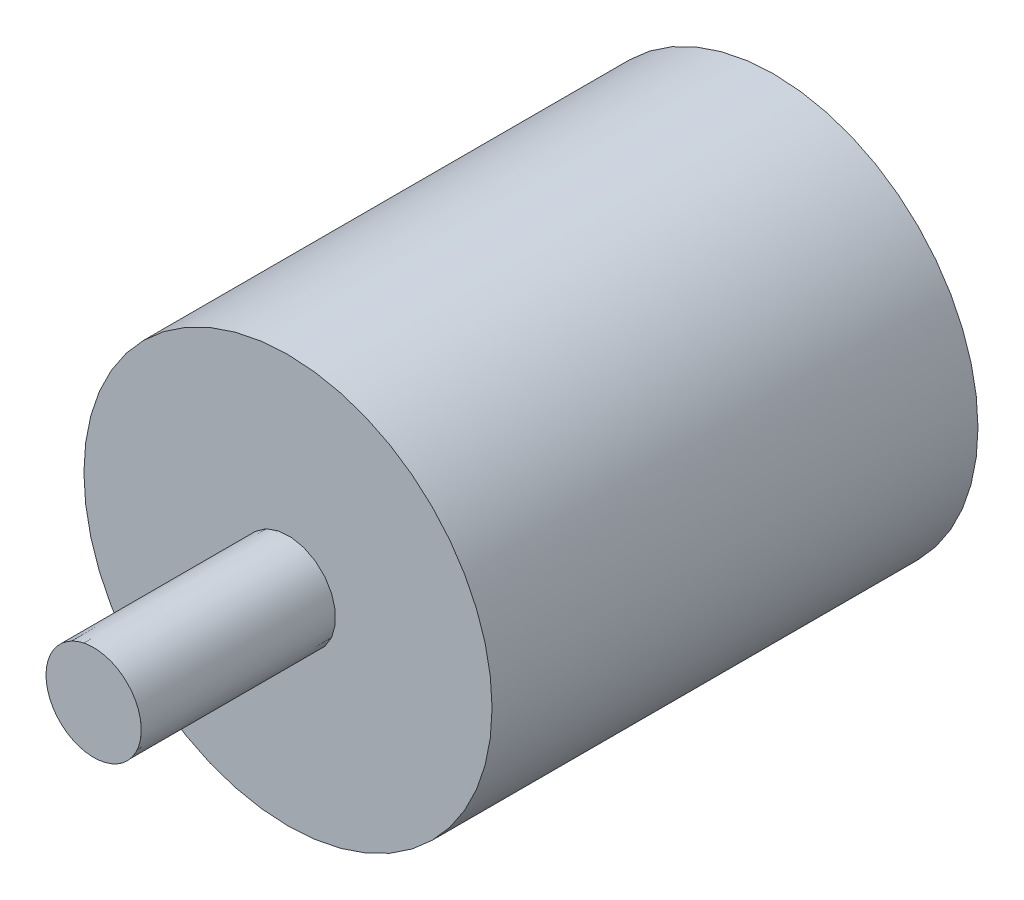
# Autodesk Inventor part: motor
Saved by Autodesk Inventor 2022 (Build 260153000, 153)
## iProperties
Created: 2022-03-03
Part Number: motor
Material: Generic
Document SubType Name: Modeling
Designer: katha
Density: 1 g/cm^3
Appearance: Default
Author: katha
Autodesk Inventor part; units mm, degrees
ref_plane "YZ Plane" through (0, 0, 0) normal (1, 0, 0) x (0, 1, 0)
ref_plane "XZ Plane" through (0, 0, 0) normal (0, 1, 0) x (-1, 0, 0)
ref_plane "XY Plane" through (0, 0, 0) normal (0, 0, 1) x (1, 0, 0)
ref_plane "Work Plane1" through (101.6836, 1.1964, 12.7076) normal (0, 0, -1) x (-1, 0, 0)
sketch "Sketch1" plane through (101.6836, 1.1964, 12.7076) normal (0, 0, -1) x (-1, 0, 0)
  circle A0 centre (0, 0) radius 2.45
  point P0 (101.6836, -1.1964)
  dimension "d0" = 4.9
  constraints: 1 centre point
  measures "d0" diameter of A0
extrude "Extrusion1" add sketch "Sketch1" along normal blind 1 and the other way blind 9
sketch "Sketch2" plane through (101.6836, 1.1964, 11.7076) normal (0, 0, -1) x (-1, 0, 0)
  circle A0 centre (0, 0) radius 2.45 projected
  circle A1 centre (0, 0) radius 10.5
  point P0 (101.6836, -1.1964)
  dimension "d5" = 21
  constraints: 1 centre point, 1 coincident
  measures "d5" diameter of A1
extrude "Extrusion2" add sketch "Sketch2" along normal blind 25 contours A0 | A1
body "Solid1"
